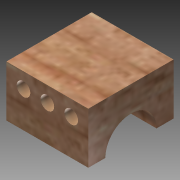
# Autodesk Inventor part: Y_RodClam_Bed
Saved by Autodesk Inventor 2014 (Build 180170000, 170)
## iProperties
Created: 2013-12-17
Part Number: Y_RodClam_Bed
Material: Birch
Document SubType Name: Modeling
Designer: Bram
Density: 0.512 g/cm^3
Appearance: Birch - Natural Medium Gloss
Author: Bram
Autodesk Inventor part; units mm, degrees
ref_plane "YZ Plane" through (0, 0, 0) normal (1, 0, 0) x (0, 1, 0)
ref_plane "XZ Plane" through (0, 0, 0) normal (0, 1, 0) x (-1, 0, 0)
ref_plane "XY Plane" through (0, 0, 0) normal (0, 0, 1) x (1, 0, 0)
sketch "Sketch1" plane through (0, 0, 0) normal (1, 0, 0) x (0, 1, 0)
  arc A0 (7.5, 0) -> (-7.5, 0) centre (0, 0) ccw
  line L0 (7.5, 0) -> (12.5, 0)
  line L1 (12.5, 0) -> (12.5, 15)
  line L2 (12.5, 15) -> (-12.5, 15)
  line L3 (-12.5, 15) -> (-12.5, 0)
  line L4 (-12.5, 0) -> (-7.5, 0)
  dimension "d0" = 15
  dimension "d1" = 12.5
  dimension "d2" = 15
  dimension "d3" = 25
  constraints: 10 end point, 2 parallel, 2 point on circle, 1 centre point, 1 coincident, 1 collinear, 1 horizontal, 1 perpendicular
  measures "d0" diameter of A0
  measures "d1" distance of A0.centre L0.end
  measures "d2" distance of L0.end L1.end
  measures "d3" distance of L1.end L2.end
extrude "Extrusion1" add sketch "Sketch1" along normal blind 24
sketch "Sketch2" plane through (0, -12.5, 0) normal (0, -1, 0) x (1, 0, 0)
  circle A0 centre (5, 10.5) radius 2
  circle A1 centre (12, 10.5) radius 2
  circle A2 centre (19, 10.5) radius 2
  dimension "d11" = 4
  constraints: 3 centre point
  measures "d11" diameter of A2
extrude "Extrusion2" cut sketch "Sketch2" against normal blind 25
body "Solid1"
